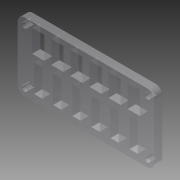
# Autodesk Inventor part: AcrylicUpperTop
Saved by Autodesk Inventor 2014 SP1 (Build 180222100, 222)
## iProperties
Created: 2016-03-18
Part Number: AcrylicUpperTop
Material: Acrylic, Clear
Document SubType Name: Modeling
Designer: Tyler
Density: 1.19 g/cm^3
Appearance: Transparent - Clear
Author: Tyler
Autodesk Inventor part; units mm, degrees
ref_plane "YZ Plane" through (0, 0, 0) normal (1, 0, 0) x (0, 1, 0)
ref_plane "XZ Plane" through (0, 0, 0) normal (0, 1, 0) x (-1, 0, 0)
ref_plane "XY Plane" through (0, 0, 0) normal (0, 0, 1) x (1, 0, 0)
sketch "Sketch1" plane through (0, 0, 0) normal (0, 1, 0) x (-1, 0, 0)
  line L0 (50, 25) -> (-50, 25)
  line L1 (-50, 25) -> (-50, -25)
  line L2 (-50, -25) -> (50, -25)
  line L3 (50, -25) -> (50, 25)
  line L4 (50, 25) -> (-50, -25) construction
  line L5 (-50, 25) -> (50, -25) construction
  point P0 (0, 0)
  dimension "d0" = 100
  dimension "d1" = 50
  constraints: 12 end point, 2 midpoint, 2 parallel, 1 horizontal, 1 perpendicular
  measures "d0" distance of L2.end L1.end
  measures "d1" distance of L1.end L0.end
extrude "Extrusion1" add sketch "Sketch1" along normal blind 6
fillet "Fillet1" radius 5 4 edges at (50, 3, 25) (50, 3, -25) (-50, 3, -25) (-50, 3, 25)
sketch "Sketch2" plane through (0, 6, 0) normal (0, 1, 0) x (1, 0, 0)
  line L0 (-39.5, -21.25) -> (-30.5, -21.25)
  line L1 (-30.5, -21.25) -> (-30.5, -4.75)
  line L2 (-30.5, -4.75) -> (-39.5, -4.75)
  line L3 (-39.5, -4.75) -> (-39.5, -21.25)
  line L4 (-39.5, -21.25) -> (-30.5, -4.75) construction
  line L5 (-30.5, -21.25) -> (-39.5, -4.75) construction
  line L6 (-25.5, -21.25) -> (-16.5, -21.25)
  line L7 (-16.5, -21.25) -> (-16.5, -4.75)
  line L8 (-16.5, -4.75) -> (-25.5, -4.75)
  line L9 (-25.5, -4.75) -> (-25.5, -21.25)
  line L10 (-25.5, -21.25) -> (-16.5, -4.75) construction
  line L11 (-16.5, -21.25) -> (-25.5, -4.75) construction
  line L12 (-11.5, -21.25) -> (-2.5, -21.25)
  line L13 (-2.5, -21.25) -> (-2.5, -4.75)
  line L14 (-2.5, -4.75) -> (-11.5, -4.75)
  line L15 (-11.5, -4.75) -> (-11.5, -21.25)
  line L16 (-11.5, -21.25) -> (-2.5, -4.75) construction
  line L17 (-2.5, -21.25) -> (-11.5, -4.75) construction
  line L18 (2.5, -21.25) -> (11.5, -21.25)
  line L19 (11.5, -21.25) -> (11.5, -4.75)
  line L20 (11.5, -4.75) -> (2.5, -4.75)
  line L21 (2.5, -4.75) -> (2.5, -21.25)
  line L22 (2.5, -21.25) -> (11.5, -4.75) construction
  line L23 (11.5, -21.25) -> (2.5, -4.75) construction
  line L24 (16.5, -21.25) -> (25.5, -21.25)
  line L25 (25.5, -21.25) -> (25.5, -4.75)
  line L26 (25.5, -4.75) -> (16.5, -4.75)
  line L27 (16.5, -4.75) -> (16.5, -21.25)
  line L28 (16.5, -21.25) -> (25.5, -4.75) construction
  line L29 (25.5, -21.25) -> (16.5, -4.75) construction
  line L30 (30.5, -21.25) -> (39.5, -21.25)
  line L31 (39.5, -21.25) -> (39.5, -4.75)
  line L32 (39.5, -4.75) -> (30.5, -4.75)
  line L33 (30.5, -4.75) -> (30.5, -21.25)
  line L34 (30.5, -21.25) -> (39.5, -4.75) construction
  line L35 (39.5, -21.25) -> (30.5, -4.75) construction
  line L36 (-45, -25) -> (45, -25) projected
  line L37 (-50, 20) -> (-50, -20) projected
  point P0 (0, 0)
  point P1 (-35, -13)
  point P2 (-21, -13)
  point P3 (-7, -13)
  point P4 (7, -13)
  point P5 (21, -13)
  point P6 (35, -13)
  dimension "d5" = 9
  dimension "d6" = 16.5
  dimension "d9" = 14
  dimension "d14" = 7
  dimension "d15" = 13
  dimension "d44" = 12
  dimension "d45" = 15
  constraints: 72 end point, 12 midpoint, 2 horizontal, 2 parallel, 1 collinear, 1 perpendicular, 54 other
  measures "d5" distance of L1.end L2.end
  measures "d6" distance of L0.end L1.end
  measures "d9" distance of L0.end L7.start
  measures "d14" horizontal distance of point (7, -13) point (0, 0)
  measures "d15" vertical distance of point (7, -13) point (0, 0)
  measures "d44" distance from line of L36 point (-35, -13)
  measures "d45" distance from line of point (-35, -13) L37
extrude "Extrusion2" cut sketch "Sketch2" against normal blind 10
sketch "Sketch3" plane through (0, 6, 0) normal (0, 1, 0) x (1, 0, 0)
  line L0 (-16.5, -21.25) -> (-25.5, -21.25) projected
  line L1 (-45, -25) -> (45, -25) projected
  line L2 (45, 25) -> (-45, 25) projected
  line L3 (-38, 0) -> (-32, 0)
  line L4 (-32, 0) -> (-32, 20)
  line L5 (-32, 20) -> (-38, 20)
  line L6 (-38, 20) -> (-38, 0)
  line L7 (-38, 0) -> (-32, 20) construction
  line L8 (-32, 0) -> (-38, 20) construction
  line L9 (-24, 0) -> (-18, 0)
  line L10 (-18, 0) -> (-18, 20)
  line L11 (-18, 20) -> (-24, 20)
  line L12 (-24, 20) -> (-24, 0)
  line L13 (-24, 0) -> (-18, 20) construction
  line L14 (-18, 0) -> (-24, 20) construction
  line L15 (-10, 0) -> (-4, 0)
  line L16 (-4, 0) -> (-4, 20)
  line L17 (-4, 20) -> (-10, 20)
  line L18 (-10, 20) -> (-10, 0)
  line L19 (-10, 0) -> (-4, 20) construction
  line L20 (-4, 0) -> (-10, 20) construction
  line L21 (4, 0) -> (10, 0)
  line L22 (10, 0) -> (10, 20)
  line L23 (10, 20) -> (4, 20)
  line L24 (4, 20) -> (4, 0)
  line L25 (4, 0) -> (10, 20) construction
  line L26 (10, 0) -> (4, 20) construction
  line L27 (18, 0) -> (24, 0)
  line L28 (24, 0) -> (24, 20)
  line L29 (24, 20) -> (18, 20)
  line L30 (18, 20) -> (18, 0)
  line L31 (18, 0) -> (24, 20) construction
  line L32 (24, 0) -> (18, 20) construction
  line L33 (32, 0) -> (38, 0)
  line L34 (38, 0) -> (38, 20)
  line L35 (38, 20) -> (32, 20)
  line L36 (32, 20) -> (32, 0)
  line L37 (32, 0) -> (38, 20) construction
  line L38 (38, 0) -> (32, 20) construction
  line L39 (-50, 20) -> (-50, -20) projected
  point P0 (0, 0)
  point P1 (-35, 10)
  point P2 (-21, 10)
  point P3 (-7, 10)
  point P4 (7, 10)
  point P5 (21, 10)
  point P6 (35, 10)
  dimension "d20" = 14
  dimension "d25" = 7
  dimension "d26" = 6
  dimension "d27" = 20
  dimension "d28" = 5
  dimension "d29" = 3.75
  dimension "d41" = 15
  dimension "d42" = 15
  dimension "d43" = 35
  constraints: 72 end point, 12 midpoint, 2 horizontal, 2 parallel, 1 collinear, 1 perpendicular, 54 other
  measures "d20" distance of L3.start L9.start
  measures "d25" horizontal distance of point (-7, 10) point (0, 0)
  measures "d26" distance of L4.end L5.end
  measures "d27" distance between parallel lines of L5 L3
  measures "d28" distance between parallel lines of L11 L2
  measures "d29" distance between parallel lines of L1 L0
  measures "d41" distance from line of point (-7, 10) L2
  measures "d42" distance from line of L39 point (-35, 10)
  measures "d43" distance from line of L1 point (-35, 10)
extrude "Extrusion3" cut sketch "Sketch3" against normal blind 10
sketch "Sketch4" plane through (0, 6, 0) normal (0, 1, 0) x (1, 0, 0)
  arc A0 (-50, -20) -> (-45, -25) centre (-45, -20) ccw projected
  arc A1 (45, -25) -> (50, -20) centre (45, -20) ccw projected
  arc A2 (50, 20) -> (45, 25) centre (45, 20) ccw projected
  arc A3 (-45, 25) -> (-50, 20) centre (-45, 20) ccw projected
  line L0 (45, 25) -> (-45, 25) projected
  line L1 (-50, 20) -> (-50, -20) projected
  point P0 (0, 0)
  dimension "d39" = 5
  dimension "d40" = 5
  constraints: 4 coincident
  measures "d39" distance from line of L1 A3.centre
  measures "d40" distance from line of A3.centre L0
hole "Hole1" at (-45, 6, -20) at (45, 6, -20) at (45, 6, 20) at (-45, 6, 20) direction (0, -1, 0) diameter 4 end through all
equation "\"d14\" = 0.5 * d9"
equation "\"d25\" = 0.5 * d20"
body "Solid1"
